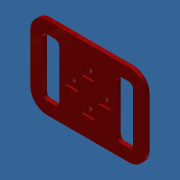
# Autodesk Inventor part: extender-plate
Saved by Autodesk Inventor 2015 (Build 190159000, 159)
## iProperties
Created: 2019-02-17
Part Number: extender-plate
Material: Generic
Document SubType Name: Modeling
Designer: gabriel
Density: 1 g/cm^3
Appearance: Default
Author: gabriel
Autodesk Inventor part; units mm, degrees
ref_plane "YZ Plane" through (0, 0, 0) normal (1, 0, 0) x (0, 1, 0)
ref_plane "XZ Plane" through (0, 0, 0) normal (0, 1, 0) x (-1, 0, 0)
ref_plane "XY Plane" through (0, 0, 0) normal (0, 0, 1) x (1, 0, 0)
sketch "Sketch2" plane through (0, 0, 0) normal (0, 0, 1) x (1, 0, 0)
  line L0 (0, 31.75) -> (44.45, 31.75)
  line L1 (44.45, 31.75) -> (44.45, 0)
  line L2 (44.45, 0) -> (0, 0)
  line L3 (0, 0) -> (0, 31.75)
  circle A0 centre (22.225, 22.225) radius 0.7937
  circle A1 centre (22.225, 9.525) radius 0.7937
  circle A2 centre (28.575, 15.875) radius 0.7937
  circle A3 centre (15.875, 15.875) radius 0.7937
  line L4 (4.7625, 26.9875) -> (11.1125, 26.9875)
  line L5 (11.1125, 26.9875) -> (11.1125, 4.7625)
  line L6 (11.1125, 4.7625) -> (4.7625, 4.7625)
  line L7 (4.7625, 4.7625) -> (4.7625, 26.9875)
  line L8 (33.3375, 26.9875) -> (39.6875, 26.9875)
  line L9 (39.6875, 26.9875) -> (39.6875, 4.7625)
  line L10 (39.6875, 4.7625) -> (33.3375, 4.7625)
  line L11 (33.3375, 4.7625) -> (33.3375, 26.9875)
  dimension "d9" = 44.45
  dimension "d10" = 31.75
  dimension "d11" = 1.5875
  dimension "d12" = 1.5875
  dimension "d13" = 1.5875
  dimension "d14" = 1.5875
  dimension "d15" = 12.7
  dimension "d16" = 12.7
  dimension "d17" = 15.875
  dimension "d18" = 22.225
  dimension "d21" = 6.35
  dimension "d22" = 6.35
  dimension "d26" = 4.7625
  dimension "d27" = 4.7625
  dimension "d28" = 4.7625
  dimension "d29" = 4.7625
  dimension "d30" = 4.7625
  dimension "d31" = 4.7625
  constraints: 24 end point, 6 parallel, 4 centre point, 3 horizontal, 3 perpendicular, 2 point on line, 1 coincident, 1 horizontal alignment, 1 vertical alignment
  measures "d9" distance of L1.end L2.end
  measures "d10" distance of L0.end L1.end
  measures "d11" diameter of A2
  measures "d12" diameter of A1
  measures "d13" diameter of A3
  measures "d14" diameter of A0
  measures "d15" distance of A2.centre A3.centre
  measures "d16" distance of A1.centre A0.centre
  measures "d17" distance from line of L0 A2.centre
  measures "d18" distance from line of L1 A1.centre
  measures "d21" horizontal distance of A2.centre A0.centre
  measures "d22" horizontal distance of A2.centre A0.centre
  measures "d26" distance between parallel lines of L0 L8
  measures "d27" distance between parallel lines of L2 L10
  measures "d28" distance between parallel lines of L1 L9
  measures "d29" distance from line of L11 A2.centre
  measures "d30" distance between parallel lines of L3 L7
  measures "d31" distance from line of L5 A3.centre
extrude "Extrusion4" add sketch "Sketch2" along normal blind 1.5875
fillet "Fillet2" radius 6.35 4 edges at (0, 31.75, 0.7937) (0, 0, 0.7937) (44.45, 0, 0.7937) (44.45, 31.75, 0.7937)
fillet "Fillet3" radius 1.5875 8 edges at (4.7625, 4.7625, 0.7937) (11.1125, 4.7625, 0.7937) (33.3375, 4.7625, 0.7937) (4.7625, 26.9875, 0.7937) (11.1125, 26.9875, 0.7937) (39.6875, 26.9875, 0.7937) (33.3375, 26.9875, 0.7937) (39.6875, 4.7625, 0.7937)
sketch "Sketch3" plane through (0, 0, 1.5875) normal (0, 0, 1) x (1, 0, 0)
  line L0 (13.4937, 18.2563) -> (18.2562, 18.2563)
  line L1 (18.2562, 18.2563) -> (18.2562, 13.4938)
  line L2 (18.2562, 13.4938) -> (13.4937, 13.4938)
  line L3 (13.4937, 13.4938) -> (13.4937, 18.2563)
  circle A0 centre (15.875, 15.875) radius 0.7937 projected
  line L4 (19.8437, 24.6063) -> (24.6062, 24.6063)
  line L5 (24.6062, 24.6063) -> (24.6062, 19.8438)
  line L6 (24.6062, 19.8438) -> (19.8437, 19.8438)
  line L7 (19.8437, 19.8438) -> (19.8437, 24.6063)
  line L8 (26.1937, 18.2563) -> (30.9562, 18.2563)
  line L9 (30.9562, 18.2563) -> (30.9562, 13.4938)
  line L10 (30.9562, 13.4938) -> (26.1937, 13.4938)
  line L11 (26.1937, 13.4938) -> (26.1937, 18.2563)
  line L12 (19.8437, 11.9063) -> (24.6062, 11.9063)
  line L13 (24.6062, 11.9063) -> (24.6062, 7.1438)
  line L14 (24.6062, 7.1438) -> (19.8437, 7.1438)
  line L15 (19.8437, 7.1438) -> (19.8437, 11.9063)
  circle A1 centre (22.225, 22.225) radius 0.7937 projected
  circle A2 centre (28.575, 15.875) radius 0.7937 projected
  circle A3 centre (22.225, 9.525) radius 0.7937 projected
  point P0 (0, 0)
  dimension "d36" = 4.7625
  dimension "d37" = 2.3813
  dimension "d38" = 2.3813
  dimension "d39" = 4.7625
  dimension "d41" = 2.3813
  dimension "d42" = 2.3813
  dimension "d43" = 2.3813
  dimension "d44" = 2.3813
  dimension "d45" = 2.3813
  dimension "d46" = 2.3813
  constraints: 32 end point, 8 parallel, 6 equal length, 4 horizontal, 4 perpendicular
  measures "d36" distance of L1.end L2.end
  measures "d37" distance from line of L3 A0.centre
  measures "d38" distance from line of A0.centre L2
  measures "d39" distance of L8.start L8.end
  measures "d41" distance from line of L7 A1.centre
  measures "d42" distance from line of A2.centre L11
  measures "d43" distance from line of L15 A3.centre
  measures "d44" distance from line of L12 A3.centre
  measures "d45" distance from line of L8 A2.centre
  measures "d46" distance from line of L4 A1.centre
extrude "Extrusion6" cut sketch "Sketch3" against normal blind 0.7937
equation "\"d12\" = d11"
equation "\"d13\" = d11"
equation "\"d14\" = d11"
equation "\"d17\" = 0.5 * d10"
equation "\"d18\" = 0.5 * d9"
equation "\"d28\" = d30"
equation "\"d29\" = d31"
equation "\"d37\" = 0.5 * d36"
equation "\"d38\" = 0.5 * d36"
equation "\"d39\" = d36"
equation "\"d41\" = d37"
equation "\"d42\" = d41"
equation "\"d43\" = d37"
equation "\"d44\" = d37"
equation "\"d45\" = d37"
equation "\"d46\" = d37"
body "Solid4"
